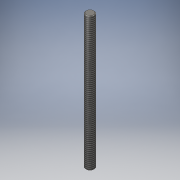
# Autodesk Inventor part: barra roscada 100 mm rosca 1 quarto
Saved by Autodesk Inventor 2019.4 (Build 234330000, 330)
## iProperties
Created: 2021-03-22
Part Number: barra roscada 100 mm rosca 1 quarto
Material: Aço, carbono
Document SubType Name: Modeling
Designer: Lattes
Density: 7.85 g/cm^3
Appearance: Semipolido
Author: Lattes
Autodesk Inventor part; units mm, degrees
ref_plane "YZ Plane" through (0, 0, 0) normal (1, 0, 0) x (0, 1, 0)
ref_plane "XZ Plane" through (0, 0, 0) normal (0, 1, 0) x (-1, 0, 0)
ref_plane "XY Plane" through (0, 0, 0) normal (0, 0, 1) x (1, 0, 0)
sketch "Esboço1" plane through (0, 0, 0) normal (0, 1, 0) x (-1, 0, 0)
  circle A0 centre (0, 0) radius 3.175
  dimension "d0" = 6.35
  constraints: 1 centre point, 1 coincident
  measures "d0" diameter of A0
extrude "Extrusão1" add sketch "Esboço1" along normal blind 100
thread "Rosca2" size "1/4-20 UNC" class "2A" standard "ANSI Unified Screw Threads" full length
chamfer "Chanfro1" distance 0.5 angle 45 2 edges at (3.175, 100, 0) (3.175, 0, 0)
